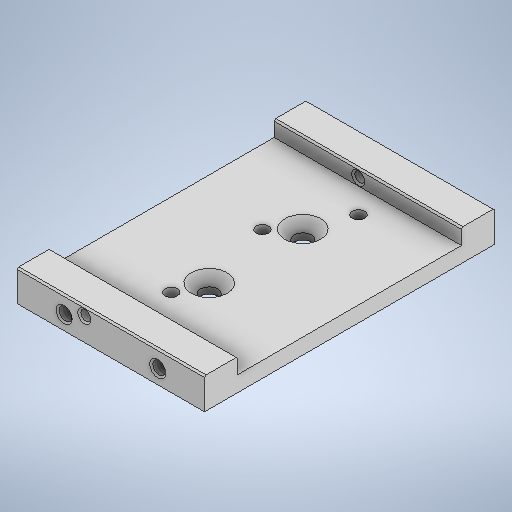
# Autodesk Inventor part: TS_V1_Fallmagazin_Wandung_int
Saved by Autodesk Inventor 2025.2 (Build 292293000, 293)
## iProperties
Created: 2025-06-10
Part Number: TS_V1_Fallmagazin_Wandung_int
Material: Generisch
Document SubType Name: Modeling
Designer: tino
Density: 1 g/cm^3
Appearance: Vorgabe
Author: tino
Autodesk Inventor part; units mm, degrees
ref_plane "YZ Plane" through (0, 0, 0) normal (1, 0, 0) x (0, 1, 0)
ref_plane "XZ Plane" through (0, 0, 0) normal (0, 1, 0) x (-1, 0, 0)
ref_plane "XY Plane" through (0, 0, 0) normal (0, 0, 1) x (1, 0, 0)
sketch "Skizze1" plane through (0, 0, 0) normal (0, 0, 1) x (1, 0, 0)
  arc A0 (-7.9107, 24.207) -> (-7.9109, 20.407) centre (-6.0635, 22.307) ccw
  line L0 (-7.9107, 24.207) -> (-4.2161, 24.2069)
  arc A1 (-4.2163, 20.4069) -> (-4.2161, 24.2069) centre (-6.0635, 22.307) ccw
  line L1 (-4.2163, 20.4069) -> (-7.9109, 20.407)
  spline S0 degree 3 poles (4.1682, 35.1897) (1.1905, 36.4598) (-2.2497, 35.1642) (-6.255, 34.1582) (-11.7361, 32.1479) (-17.2675, 27.437) (-17.3979, 22.2805) (-19.1794, 11.8373) (-24.2043, -4.2198) (-21.9122, -21.3619) (-15.7263, -32.1361) (-8.9601, -34.8731) (-7.7344, -35.2068) knots 0 0 0 0 0.05535 0.076528 0.211782 0.295547 0.382964 0.432922 0.754884 0.81234 0.967238 1 1 1 1
  spline S1 degree 3 poles (-7.7344, -35.2068) (-2.4391, -36.6482) (4.9342, -35.145) (14.3889, -31.3641) (20.2206, -28.2765) (23.0847, -23.1792) (23.281, -18.9959) (17.3062, -16.4997) (13.7398, -19.2937) (6.9074, -22.9332) (-1.1986, -27.1621) (-10.3055, -22.9326) (-14.0352, -10.4002) (-9.4599, -0.926) (-6.8334, 0.3153) (-5.9182, 2.0588) (-5.9367, 4.1791) (-8.2887, 5.2306) (-8.3642, 10.4373) (-1.0106, 14.1251) (4.0821, 20.0507) (3.0635, 26.3026) (2.9493, 28.6136) (3.7888, 29.834) (5.5778, 31.0924) (6.6132, 32.7745) (5.2458, 34.7086) (4.2656, 35.1481) (4.1682, 35.1897) knots 0 0 0 0 0.14153 0.17035 0.245987 0.25892 0.290227 0.326265 0.372233 0.38898 0.482096 0.508256 0.624416 0.647418 0.715274 0.72607 0.746892 0.801722 0.811885 0.848514 0.916356 0.943374 0.948219 0.962959 0.96651 0.98188 0.998188 1 1 1 1
  line L2 (-4.2163, 20.4069) -> (-7.9109, 20.407)
  arc A2 (-4.2163, 20.4069) -> (-4.2161, 24.2069) centre (-6.0635, 22.307) ccw
  line L3 (-7.9107, 24.207) -> (-4.2161, 24.2069)
  arc A3 (-7.9107, 24.207) -> (-7.9109, 20.407) centre (-6.0635, 22.307) ccw
  line L4 (-22.9949, 35.8296) -> (22.9949, 35.8296) construction
  line L5 (22.9949, 35.8296) -> (22.9949, -35.8296) construction
  line L6 (22.9949, -35.8296) -> (-22.9949, -35.8296) construction
  line L7 (-22.9949, -35.8296) -> (-22.9949, 35.8296) construction
  line L8 (-22.9949, 35.8296) -> (22.9949, -35.8296) construction
  line L9 (-22.9949, -35.8296) -> (22.9949, 35.8296) construction
  circle A4 centre (3.8745, -36.2796) radius 1.25 construction
  line L10 (1.2146, -35.8296) -> (11.5877, -35.8296) construction
  line L11 (3.8745, -36.2796) -> (3.8745, -35.0296) construction
  circle A5 centre (4.7955, 36.2796) radius 1.25 construction
  line L12 (4.7955, 36.2796) -> (4.7955, 35.0296) construction
  line L13 (3.124, 35.8296) -> (12.547, 35.8296) construction
  point P0 (0, 0)
  point P1 (0, 0)
  point P2 (0, 0)
  dimension "d88" = 2.5
  dimension "d91" = 2.5
  dimension "d89" = 0.8
  dimension "d92" = 0.8
  constraints: 28 end point, 8 point on circle, 4 centre point, 4 perpendicular, 3 vertical, 2 collinear, 2 horizontal, 2 midpoint, 2 vertical alignment, 1 coincident, 8 other
sketch "Skizze9" plane through (0, 0, 0) normal (0, 0, 1) x (1, 0, 0)
  line L0 (-30, 42.5) -> (30, 42.5)
  line L1 (30, 42.5) -> (30, -42.5)
  line L2 (30, -42.5) -> (-30, -42.5)
  line L3 (-30, 42.5) -> (30, -42.5) construction
  line L4 (30, 42.5) -> (-30, -42.5) construction
  spline S0 degree 3 poles (4.1682, 35.1897) (1.1905, 36.4598) (-2.2497, 35.1642) (-6.255, 34.1582) (-11.7361, 32.1479) (-17.2675, 27.437) (-17.3979, 22.2805) (-19.1794, 11.8373) (-24.2043, -4.2198) (-21.9122, -21.3619) (-15.7263, -32.1361) (-8.9601, -34.8731) (-7.7344, -35.2068) knots 0 0 0 0 0.05535 0.076528 0.211782 0.295547 0.382964 0.432922 0.754884 0.81234 0.967238 1 1 1 1
  spline S1 degree 3 poles (-7.7344, -35.2068) (-2.4391, -36.6482) (4.9342, -35.145) (14.3889, -31.3641) (20.2206, -28.2765) (23.0847, -23.1792) (23.281, -18.9959) (17.3062, -16.4997) (13.7398, -19.2937) (6.9074, -22.9332) (-1.1986, -27.1621) (-10.3055, -22.9326) (-14.0352, -10.4002) (-9.4599, -0.926) (-6.8334, 0.3153) (-5.9182, 2.0588) (-5.9367, 4.1791) (-8.2887, 5.2306) (-8.3642, 10.4373) (-1.0106, 14.1251) (4.0821, 20.0507) (3.0635, 26.3026) (2.9493, 28.6136) (3.7888, 29.834) (5.5778, 31.0924) (6.6132, 32.7745) (5.2458, 34.7086) (4.2656, 35.1481) (4.1682, 35.1897) knots 0 0 0 0 0.14153 0.17035 0.245987 0.25892 0.290227 0.326265 0.372233 0.38898 0.482096 0.508256 0.624416 0.647418 0.715274 0.72607 0.746892 0.801722 0.811885 0.848514 0.916356 0.943374 0.948219 0.962959 0.96651 0.98188 0.998188 1 1 1 1
  circle A0 centre (-3.5, -23.6754) radius 2
  circle A1 centre (5.0009, 27.8502) radius 2
  circle A2 centre (-6.3, 8.3754) radius 2
  line L5 (-30, -35.8296) -> (30, -35.8296)
  line L6 (-30, -42.5) -> (-30, 42.5)
  line L7 (-30, 35.8296) -> (30, 35.8296)
  point P0 (0, 0)
  point P1 (-2.7819, -35.8296)
  point P2 (1.074, 35.8296)
  dimension "d68" = 60
  dimension "d69" = 85
  dimension "d180" = 4
  dimension "d182" = 4
  dimension "d183" = 4
  dimension "d184" = 33.5
  dimension "d186" = 24.9991
  dimension "d221" = 36.3
  constraints: 16 end point, 4 point on line, 3 centre point, 3 horizontal, 3 perpendicular, 2 midpoint, 1 parallel, 1 vertical, 4 other
  measures "d68" distance of L0.start L0.end
  measures "d69" distance of L0.end L1.end
  measures "d180" diameter of A0
  measures "d182" diameter of A2
  measures "d183" diameter of A1
  measures "d184" distance from line of L1 A0.centre
  measures "d186" distance from line of L1 A1.centre
  measures "d221" distance from line of L1 A2.centre
extrude "Extrusion3" add sketch "Skizze9" along normal blind 5 contours L0 L1 L7 L6 | L5 L1 L2 L6
sketch "Skizze11" plane through (0, 0, 0) normal (0, 0, -1) x (-1, 0, 0)
  line L0 (30, -42.5) -> (-30, -42.5) projected
  line L1 (30, 42.5) -> (30, -42.5) projected
  line L2 (-30, -42.5) -> (30, -42.5)
  line L3 (30, -42.5) -> (30, 42.5)
  line L4 (30, 42.5) -> (-30, 42.5)
  line L5 (-30, 42.5) -> (-30, -42.5)
  point P0 (0, 0)
  constraints: 8 end point, 2 parallel, 1 horizontal, 1 perpendicular
extrude "Extrusion4" add sketch "Skizze11" along normal blind 1.5
chamfer "Fasen2" distance 0.5 angle 45 2 edges at (0, -35.8296, 5) (0, 35.8296, 5)
sketch "Skizze15" plane through (-30, 42.5, 5) normal (0, 1, 0) x (1, 0, 0)
  line L0 (60, 0) -> (0, 0) projected
  line L1 (0, 6.5) -> (60, 6.5) projected
  line L2 (60, 0) -> (0, 0)
  line L3 (0, 0) -> (0, 6.5)
  line L4 (0, 6.5) -> (60, 6.5)
  line L5 (60, 6.5) -> (60, 0)
  point P0 (30, 5)
  constraints: 8 end point, 2 parallel, 1 horizontal, 1 perpendicular
extrude "Extrusion6" add sketch "Skizze15" along normal blind 4
sketch "Skizze16" plane through (-30, -42.5, 5) normal (0, -1, 0) x (1, 0, 0)
  line L0 (0, -6.5) -> (0, 0) projected
  line L1 (60, -6.5) -> (0, -6.5) projected
  line L2 (0, 0) -> (60, 0)
  line L3 (60, 0) -> (60, -6.5)
  line L4 (60, -6.5) -> (0, -6.5)
  line L5 (0, -6.5) -> (0, 0)
  point P0 (30, -5)
  constraints: 8 end point, 2 parallel, 1 horizontal, 1 perpendicular
extrude "Extrusion7" add sketch "Skizze16" along normal blind 4
sketch "Skizze17" plane through (0, 0, -1.5) normal (0, 0, -1) x (-1, 0, 0)
  line L0 (30, 46.5) -> (30, -46.5) projected
  line L1 (-30, 46.5) -> (30, 46.5) projected
  line L2 (-30, -46.5) -> (-30, 46.5) projected
  line L3 (30, -46.5) -> (-30, -46.5) projected
  point P0 (0, 0)
extrude "Extrusion8" add sketch "Skizze17" along normal blind 3.5
chamfer "Fasen4" distance 0.5 angle 45 2 edges at (0, 46.5, 5) (0, -46.5, 5)
sketch "Skizze20" plane through (0, 0, 0) normal (0, 0, 1) x (1, 0, 0)
  line L0 (-30, -46.5) -> (30, -46.5) projected
  line L1 (30, 35.8296) -> (30, -35.8296) projected
  point P0 (0, 0)
  point P1 (0, -15)
  point P2 (0, 0)
  point P3 (0, 15)
  dimension "d152" = 15
  dimension "d153" = 15
  constraints: 2 vertical alignment
  measures "d152" distance of point (0, -15) point (0, 0)
  measures "d153" distance of point (0, 15) point (0, 0)
hole "Bohrung10" at (0, -15, 0) at (0, 15, 0) direction (0, 0, -1) diameter 5.5 end through all countersink diameter 11.5 countersink angle 90
sketch "Skizze21" plane through (-30, -46.5, 5) normal (0, -1, 0) x (1, 0, 0)
  line L0 (60, -10) -> (0, -10) projected
  line L1 (60, 0) -> (0, 0) projected
  line L2 (60, -0.5) -> (60, -10) projected
  line L3 (0, -0.5) -> (0, -10) projected
  point P0 (30, -5)
  point P1 (15, -5.5)
  point P2 (45, -5.5)
  point P3 (60, -5.25)
  dimension "d161" = 10
  dimension "d163" = 60
  dimension "d164" = 15
  dimension "d165" = 15
  dimension "d179" = 4.5
  constraints: 1 horizontal alignment, 1 midpoint
  measures "d161" distance between parallel lines of L0 L1
  measures "d163" distance between parallel lines of L2 L3
  measures "d164" distance from line of L3 point (15, -5.5)
  measures "d165" horizontal distance of point (60, -5.25) point (45, -5.5)
  measures "d179" distance from line of L0 point (15, -5.5)
hole "Bohrung11" at (15, -46.5, -0.5) at (-15, -46.5, -0.5) direction (0, 1, 0) diameter 4.134 depth 6 tip angle 118 thread size "M5x0.8" class "6H" standard "ISO Metric profile"
chamfer "Fasen5" distance 0.5 angle 45 2 edges at (-15, -46.5, 1.567) (15, -46.5, 1.567)
mirror "Spiegeln4" about plane through (0, 0, 0) normal (0, 1, 0) of "Bohrung11"
chamfer "Fasen6" distance 0.5 angle 45 2 edges at (15, 46.5, 1.567) (-15, 46.5, 1.567)
sketch "Skizze22" plane through (0, 0, 0) normal (0, 0, 1) x (1, 0, 0)
  circle A0 centre (-8.5268, -36.2796) radius 1.25 construction
  line L0 (30, -35.8296) -> (-30, -35.8296) construction
  line L1 (-19.0292, -35.0296) -> (-13.2341, -35.0296) construction
  spline S0 degree 3 poles (4.1682, 35.1897) (1.1905, 36.4598) (-2.2497, 35.1642) (-6.255, 34.1582) (-11.7361, 32.1479) (-17.2675, 27.437) (-17.3979, 22.2805) (-19.1794, 11.8373) (-24.2043, -4.2198) (-21.9122, -21.3619) (-15.7263, -32.1361) (-8.9601, -34.8731) (-7.7344, -35.2068) knots 0 0 0 0 0.05535 0.076528 0.211782 0.295547 0.382964 0.432922 0.754884 0.81234 0.967238 1 1 1 1 construction
  circle A1 centre (-3.0739, 36.2796) radius 1.25 construction
  line L2 (-18.7054, 35.0296) -> (-14.3963, 35.0296) construction
  line L3 (-30, 35.8296) -> (30, 35.8296) construction
  point P0 (0, 0)
  dimension "d188" = 2.5
  dimension "d189" = 0.8
  dimension "d190" = 2.5
  dimension "d191" = 0.8
  constraints: 4 end point, 2 centre point, 2 horizontal, 2 tangent, 2 other
  measures "d188" diameter of A0
  measures "d189" distance between parallel lines of L0 L1
  measures "d190" diameter of A1
  measures "d191" distance between parallel lines of L3 L2
sketch "Skizze23" plane through (-30, -35.8296, 0) normal (0, 1, 0) x (1, 0, 0)
  line L0 (20.2232, 0) -> (22.7232, 0) construction
  line L1 (0, -5) -> (60, -5) projected
  line L2 (60, -4.5) -> (0, -4.5) projected
  line L3 (60, 0) -> (0, 0) projected
  point P0 (30, 0)
  point P1 (21.4732, -2.25)
  point P2 (21.4732, 0)
  dimension "d218" = 4.5
  dimension "d219" = 2.25
  constraints: 1 midpoint, 1 vertical alignment
  measures "d218" distance between parallel lines of L2 L3
  measures "d219" distance from line of L3 point (21.473, -2.25)
hole "Bohrung12" at (-8.5268, -35.8296, 2.25) direction (0, -1, 0) diameter 3.242 end through all thread size "M4x0.7" class "6H" standard "ISO Metric profile"
chamfer "Fasen7" distance 0.5 angle 45 2 edges at (-8.5268, -35.8296, 0.629) (-8.5268, -46.5, 0.629)
sketch "Skizze24" plane through (-30, 35.8296, 0) normal (0, -1, 0) x (1, 0, 0)
  line L0 (28.1761, 0) -> (25.6761, 0) construction
  line L1 (60, 5) -> (0, 5) projected
  line L2 (0, 0) -> (60, 0) projected
  line L3 (0, 4.5) -> (60, 4.5) projected
  point P0 (30, 0)
  point P1 (26.9261, 2.25)
  point P2 (26.9261, 0)
  dimension "d205" = 2.25
  dimension "d220" = 4.5
  constraints: 1 midpoint, 1 vertical alignment
  measures "d205" distance from line of point (26.926, 2.25) L2
  measures "d220" distance between parallel lines of L3 L2
hole "Bohrung13" at (-3.0739, 35.8296, 2.25) direction (0, 1, 0) diameter 3.242 end through all thread size "M4x0.7" class "6H" standard "ISO Metric profile"
chamfer "Fasen8" distance 0.5 angle 45 2 edges at (-3.0739, 35.8296, 3.871) (-3.0739, 46.5, 3.871)
extrude "Extrusion10" cut sketch "Skizze9" against normal blind 3 contours A0 | A2 | A1
equation "\"d91\" = Kugeldurchmesser"
equation "\"d89\" = Kugelhoehe"
equation "\"d92\" = Kugelhoehe"
equation "\"d68\" = Breite_innen"
equation "\"d69\" = Laenge_innen"
equation "\"d152\" = Anbindung_Kolben"
equation "\"d153\" = d152"
equation "\"d191\" = d189"
equation "\"Breite_innen\" = 60"
equation "\"Laenge_innen\" = 85"
equation "\"Laenge_aussen\" = Laenge_innen + 2 * Wanddicke"
equation "\"Absatz\" = 2"
equation "\"Kugeldurchmesser\" = 2.5"
equation "\"Kugelhoehe\" = 0.8"
equation "\"Anbindung_Kolben\" = 15"
equation "\"Wanddicke\" = 10"
